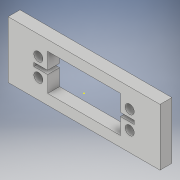
# Autodesk Inventor part: Cou-Bon
Saved by Autodesk Inventor 2018 (Build 220112000, 112)
## iProperties
Created: 2018-02-13
Part Number: Cou-Bon
Material: Generic
Document SubType Name: Modeling
Designer: Lilia
Density: 1 g/cm^3
Appearance: Default
Author: Lilia
Autodesk Inventor part; units mm, degrees
ref_plane "YZ Plane" through (0, 0, 0) normal (1, 0, 0) x (0, 1, 0)
ref_plane "XZ Plane" through (0, 0, 0) normal (0, 1, 0) x (-1, 0, 0)
ref_plane "XY Plane" through (0, 0, 0) normal (0, 0, 1) x (1, 0, 0)
sketch "Sketch1" plane through (0, 0, 0) normal (0, 0, 1) x (1, 0, 0)
  line L0 (-20, 10.0166) -> (20, 10.0166)
  line L1 (19.9334, -9.9833) -> (-19.9334, -9.9833)
  line L2 (-20, 10.0166) -> (19.9334, -9.9833) construction
  line L3 (20, 10.0166) -> (-19.9334, -9.9833) construction
  line L4 (-41.6, 15.6) -> (41.6, 15.6)
  line L5 (41.6, 15.6) -> (41.6, -15.6)
  line L6 (41.6, -15.6) -> (-41.6, -15.6)
  line L7 (-41.6, -15.6) -> (-41.6, 15.6)
  line L8 (-41.6, 15.6) -> (41.6, -15.6) construction
  line L9 (41.6, 15.6) -> (-41.6, -15.6) construction
  line L10 (-20, 1.0167) -> (-27.5, 1.0167)
  line L11 (-27.5, 1.0167) -> (-27.5, -0.9833)
  line L12 (-27.5, -0.9833) -> (-19.9334, -0.9833)
  line L13 (20, 1.0167) -> (27.5, 1.0167)
  line L14 (27.5, 1.0167) -> (27.5, -0.9833)
  line L15 (27.5, -0.9833) -> (19.9334, -0.9833)
  line L16 (-20, 1.0167) -> (-20, 10.0166)
  line L17 (-19.9334, -9.9833) -> (-19.9334, -0.9833)
  line L18 (19.9334, -0.9833) -> (19.9334, -9.9833)
  line L19 (20, 1.0167) -> (20, 10.0166)
  point P0 (0, 0)
  point P1 (-27.5, 0.0167)
  point P2 (-0.0333, 0.0167)
  point P3 (0, 10.0166)
  point P4 (0, 0)
  dimension "CInt" = 40
  dimension "LInt" = 20
  dimension "Cext" = 83.2
  dimension "Lext" = 31.2
  dimension "Cpeq" = 7.5
  dimension "Lpeq" = 2
  dimension "d10" = 7.5
  dimension "d11" = 2
  constraints: 40 end point, 8 parallel, 6 midpoint, 4 horizontal, 3 perpendicular, 3 point on line, 1 horizontal alignment, 1 vertical, 1 vertical alignment
  measures "CInt" distance of L0.start L0.end
  measures "LInt" distance of L1.end L0.start
  measures "Cext" distance of L4.start L4.end
  measures "Lext" distance of L6.end L4.start
  measures "Cpeq" distance of L10.start L10.end
  measures "Lpeq" distance of L10.end L11.end
  measures "d10" distance of L13.start L13.end
  measures "d11" distance of L13.end L14.end
extrude "Extrusion1" add sketch "Sketch1" along normal mid plane 6.5
sketch "Sketch8" plane through (0, 0, 3.25) normal (0, 0, 1) x (1, 0, 0)
  point P0 (0, 0)
hole "Hole1" at (-25, 5.0167, 3.25) direction (0, 0, -1) diameter 5 end through all
pattern_linear "Rectangular Pattern1" count 2 spacing 10 along (0, -1, 0) of "Hole1"
hole "Hole2" at (25, 5.0167, 3.25) direction (0, 0, -1) diameter 5 end through all
pattern_linear "Rectangular Pattern2" count 2 spacing 10 along (0, -1, 0) of "Hole2"
body "Solid1"
